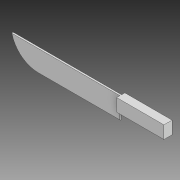
# Autodesk Inventor part: Knife
Saved by Autodesk Inventor 2020 (Build 240168000, 168)
## iProperties
Created: 2020-10-19
Part Number: Knife
Material: Generic
Document SubType Name: Modeling
Designer: DDeGo
Density: 1 g/cm^3
Appearance: Default
Author: DDeGo
Autodesk Inventor part; units mm, degrees
ref_plane "YZ Plane" through (0, 0, 0) normal (1, 0, 0) x (0, 1, 0)
ref_plane "XZ Plane" through (0, 0, 0) normal (0, 1, 0) x (-1, 0, 0)
ref_plane "XY Plane" through (0, 0, 0) normal (0, 0, 1) x (1, 0, 0)
sketch "Sketch1" plane through (0, 0, 0) normal (0, 0, 1) x (1, 0, 0)
  line L0 (0, 0) -> (-150, 0)
  line L1 (-150, 0) -> (-150, 40) construction
  line L2 (-150, 40) -> (0, 40)
  line L3 (0, 40) -> (0, 0)
  arc A0 (-200, 40) -> (-150, 0) centre (-150, 51.25) ccw
  line L4 (-200, 40) -> (-150, 40)
  dimension "d0" = 150
  dimension "d1" = 50
  dimension "d2" = 40
  constraints: 10 end point, 2 horizontal, 2 parallel, 2 point on circle, 1 centre point, 1 perpendicular, 1 tangent
  measures "d0" distance between parallel lines of L1 L3
  measures "d1" distance from line of L4.start L1
  measures "d2" distance of L2.end L0.start
extrude "Extrusion1" add sketch "Sketch1" along normal mid plane 3
sketch "Sketch2" plane through (0, 0, 0) normal (0, 0, 1) x (1, 0, 0)
  line L0 (0, 40) -> (-200, 40) projected
  line L1 (0, 40) -> (86.8358, 40)
  line L2 (86.8358, 40) -> (86.8358, 16.7298)
  line L3 (86.8358, 16.7298) -> (0, 16.7298)
  line L4 (0, 16.7298) -> (0, 40)
  point P0 (0, 0)
  constraints: 8 end point, 2 parallel, 1 horizontal, 1 perpendicular
extrude "Extrusion2" add sketch "Sketch2" along normal mid plane 15
chamfer "Chamfer1" distance 1.5 angle 45 4 edges at (-75, 0, 1.5) (-182.0156, 11.2305, 1.5) (-75, 0, -1.5) (-182.0156, 11.2305, -1.5)
body "Solid1"
